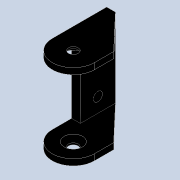
# Autodesk Inventor part: Y Axis Drag Chain Mount Bolted
Saved by Autodesk Inventor 2022 (Build 260153000, 153)
## iProperties
Created: 2021-10-29
Part Number: Y Axis Drag Chain Mount Bolted
Material: Generic
Document SubType Name: Modeling
Designer: Coy
Density: 1 g/cm^3
Appearance: Anodized - Black
Author: Coy
Autodesk Inventor part; units mm, degrees
ref_plane "YZ Plane" through (0, 0, 0) normal (1, 0, 0) x (0, 1, 0)
ref_plane "XZ Plane" through (0, 0, 0) normal (0, 1, 0) x (-1, 0, 0)
ref_plane "XY Plane" through (0, 0, 0) normal (0, 0, 1) x (1, 0, 0)
sketch "Sketch1" plane through (0, 0, 0) normal (1, 0, 0) x (0, 1, 0)
  line L0 (0, 0) -> (55, 0)
  line L1 (55, 0) -> (55, 20)
  line L2 (55, 20) -> (0, 20)
  line L3 (0, 20) -> (0, 0)
  line L4 (55, 10) -> (0, 10) construction
  circle A0 centre (40, 10) radius 2.6
  circle A1 centre (15, 10) radius 2.6
  dimension "d0" = 55
  dimension "d1" = 20
  dimension "d2" = 5.2
  dimension "d3" = 5.2
  dimension "d4" = 15
  dimension "d5" = 15
  constraints: 10 end point, 2 centre point, 2 midpoint, 2 parallel, 2 point on line, 1 horizontal, 1 perpendicular
  measures "d0" distance of L2.end L1.end
  measures "d1" distance of L1.end L0.end
  measures "d2" diameter of A0
  measures "d3" diameter of A1
  measures "d4" distance from line of L1 A0.centre
  measures "d5" distance from line of L3 A1.centre
extrude "Extrusion1" add sketch "Sketch1" along normal blind 5
sketch "Sketch2" plane through (0, 0, 20) normal (0, 0, 1) x (1, 0, 0)
  line L0 (0, 48.25) -> (29, 48.25)
  line L1 (29, 48.25) -> (29, 55)
  line L2 (29, 55) -> (0, 55)
  line L3 (0, 55) -> (0, 48.25)
  line L4 (0, 0) -> (29, 0)
  line L5 (29, 0) -> (29, 6.75)
  line L6 (29, 6.75) -> (0, 6.75)
  line L7 (0, 6.75) -> (0, 0)
  line L8 (0, 55) -> (5, 55) projected
  line L9 (0, 0) -> (0, 55) projected
  line L10 (0, 55) -> (0, 0) projected
  line L11 (0, 0) -> (5, 0) projected
  line L12 (5, 55) -> (5, 0) projected
  line L13 (0, 55) -> (5, 55) projected
  line L14 (29, 55) -> (24, 55)
  line L15 (24, 55) -> (24, 0)
  line L16 (24, 0) -> (29, 0)
  line L17 (29, 0) -> (29, 55)
  point P0 (5, 48.25)
  point P1 (5, 6.75)
  point P2 (24, 6.75)
  point P3 (24, 48.25)
  dimension "d8" = 29
  dimension "d9" = 29
  dimension "d12" = 6.75
  dimension "d13" = 41.5
  dimension "d33" = 5
  constraints: 24 end point, 6 parallel, 3 horizontal, 3 perpendicular, 2 collinear, 1 point on line
  measures "d8" distance of L1.end L2.end
  measures "d9" distance of L5.end L6.end
  measures "d12" distance of L0.end L1.end
  measures "d13" distance between parallel lines of L6 L0
  measures "d33" distance of L16.end L15.end
extrude "Extrusion2" add sketch "Sketch2" along normal blind 23 contours L3 L2 L12 L0 | L12 L2 L15 L0 | L6 L12 L4 L7 | L6 L15 L4 L12
fillet "Fillet1" radius 12 4 edges at (24, 51.625, 43) (0, 51.625, 43) (24, 3.375, 43) (0, 3.375, 43)
sketch "Sketch3" plane through (0, 55, 0) normal (0, 1, 0) x (1, 0, 0)
  circle A0 centre (12, -31) radius 2.75
  arc A1 (0, -31) -> (24, -31) centre (12, -31) ccw projected
  point P0 (0, 0)
  dimension "d17" = 5.5
  constraints: 1 centre point, 1 coincident
  measures "d17" diameter of A0
extrude "Extrusion3" cut sketch "Sketch3" against normal through all
sketch "Sketch4" plane through (0, 0, 0) normal (0, 0, -1) x (-1, 0, 0)
  line L0 (0, 55) -> (-5, 55) projected
  line L1 (0, 55) -> (-29, 55)
  line L2 (-29, 55) -> (-29, 51.75)
  line L3 (-29, 51.75) -> (0, 51.75)
  line L4 (0, 51.75) -> (0, 55)
  line L5 (0, 6.75) -> (0, 0) projected
  line L6 (-29, 0) -> (-29, 6.75) projected
  line L7 (0, 0) -> (-29, 0)
  line L8 (-29, 0) -> (-29, 3.25)
  line L9 (-29, 3.25) -> (0, 3.25)
  line L10 (0, 3.25) -> (0, 0)
  dimension "d26" = 3.25
  dimension "d27" = 3.25
  constraints: 16 end point, 4 parallel, 2 horizontal, 2 perpendicular, 1 point on line
  measures "d26" distance of L2.end L1.end
  measures "d27" distance of L7.end L8.end
extrude "Extrusion4" cut sketch "Sketch4" against normal through all
chamfer "Chamfer3" distance 2.5 angle 45 2 edges at (9.25, 48.25, 31) (9.25, 6.75, 31)
chamfer "Chamfer4" distance 20 distance2 19 1 edges at (5, 50, 20) measured on face at (5, 23.6407, 2.523)
chamfer "Chamfer5" distance 20 distance2 19 1 edges at (5, 5, 20) measured on face at (5, 22.474, 2.523)
equation "\"d3\" = d2"
equation "\"d5\" = d4"
equation "\"d9\" = d8"
body "Solid1"
